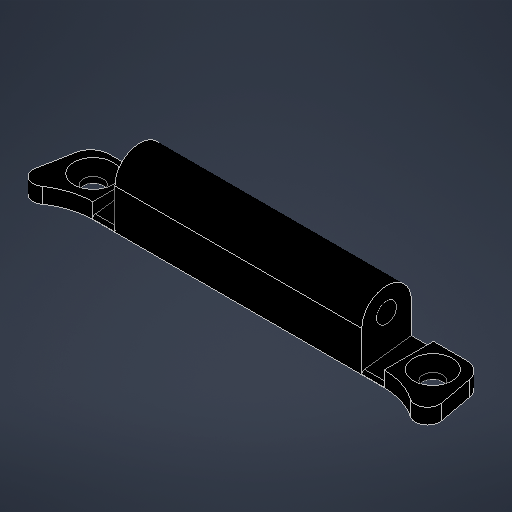
# Autodesk Inventor part: Dribbler Mount
Saved by Autodesk Inventor 2026.1 (Build 301233020, 233B)
## iProperties
Created: 2026-04-20
Part Number: Dribbler Mount
Material: Generic
Document SubType Name: Modeling
Designer: Bahaa
Mass: 3.13625 g
Surface Area: 24.6798 cm^2
Volume: 3.13625 cm^3
Density: 1 g/cm^3
Appearance: Black PLA
Author: Bahaa
Autodesk Inventor part; units mm, degrees
ref_plane "YZ Plane" through (0, 0, 0) normal (1, 0, 0) x (0, 1, 0)
ref_plane "XZ Plane" through (0, 0, 0) normal (0, 1, 0) x (-1, 0, 0)
ref_plane "XY Plane" through (0, 0, 0) normal (0, 0, 1) x (1, 0, 0)
sketch "Sketch1" plane through (0, 0, 0) normal (0, 0, 1) x (1, 0, 0)
  line L0 (-20, -4) -> (20, -4)
  line L1 (20, -4) -> (20, 4)
  line L2 (20, 4) -> (-20, 4)
  line L3 (-20, 4) -> (-20, -4)
  line L4 (-20, -4) -> (20, 4) construction
  line L5 (20, -4) -> (-20, 4) construction
  line L6 (-23.4, -4) -> (23.4, -4)
  line L7 (23.4, -4) -> (23.4, 4)
  line L8 (23.4, 4) -> (-23.4, 4)
  line L9 (-23.4, 4) -> (-23.4, -4)
  line L10 (-23.4, -4) -> (23.4, 4) construction
  line L11 (23.4, -4) -> (-23.4, 4) construction
  line L12 (-31.4, -4) -> (-23.4, -4)
  line L13 (-23.4, -4) -> (-23.4, 4)
  line L14 (-23.4, 4) -> (-28.9164, 4)
  line L15 (-31.4, 4) -> (-31.4, -4)
  circle A0 centre (-23.4, -15.5) radius 11.5
  line L16 (-31.8637, 1.5601) -> (-34.6978, -13.3529)
  line L17 (0, -4) -> (0, 4) construction
  circle A1 centre (23.4, -15.5) radius 11.5
  line L18 (31.8637, 1.5601) -> (34.6978, -13.3529)
  line L19 (31.4, -4) -> (23.4, -4)
  line L20 (23.4, 4) -> (28.9164, 4)
  line L21 (31.4, 4) -> (31.4, -4)
  line L22 (31.4, -4) -> (23.4, 4) construction
  line L23 (23.4, -4) -> (31.4, 4) construction
  arc A2 (-28.9164, 4) -> (-31.8637, 1.5601) centre (-28.9164, 1) ccw
  arc A3 (31.8637, 1.5601) -> (28.9164, 4) centre (28.9164, 1) ccw
  line L24 (23.4, -1.5) -> (-23.4, -1.5)
  line L25 (-20, 4) -> (-24, 4)
  line L26 (-24, 4) -> (-24, -4.0157)
  line L27 (-24, -4.0157) -> (-20, -4.0157)
  line L28 (-20, -4.0157) -> (-20, 4)
  line L29 (20, 4) -> (24, 4)
  line L30 (24, 4) -> (24, -4)
  line L31 (24, -4) -> (20, -4)
  line L32 (20, -4) -> (20, 4)
  point P0 (0, 0)
  point P1 (-20, 0)
  point P2 (-23.4, 0)
  point P3 (-27.5, 0)
  point P4 (27.5, 0)
  point P5 (23.4, -4)
  point P6 (-20, -1.5)
  point P7 (20, -1.5)
  point P8 (-31.4, 0)
  dimension "d0" = 40
  dimension "d1" = 8
  dimension "d3" = 3.4
  dimension "d4" = 8
  dimension "d5" = 8
  dimension "d6" = 0
  dimension "d7" = 11.5
  dimension "d8" = 23
  dimension "d11" = 3
  dimension "d31" = 5.5
  dimension "d35" = 27.5
  dimension "d40" = 4
  dimension "d41" = 4
  constraints: 62 end point, 10 midpoint, 10 parallel, 8 point on line, 7 symmetric about line, 6 perpendicular, 6 point on circle, 5 horizontal, 5 tangent, 3 centre point, 2 collinear, 1 equal radius, 1 horizontal alignment, 10 other
  measures "d0" distance of L2.end L1.end
  measures "d1" distance of L1.end L0.end
  measures "d3" distance of point (-20, 0) point (-23.4, 0)
  measures "d4" distance of L15.start L13.end
  measures "d5" distance of L15.start L12.start
  measures "d6" distance from line of L9 A0.centre
  measures "d7" vertical distance of L0.start A0.centre
  measures "d8" diameter of A0
  measures "d11" radius of A2
  measures "d31" distance from line of point (0, 4) L24
  measures "d35" distance of point (0, 0) point (-27.5, 0)
  measures "d40" distance of L27.end L26.end
  measures "d41" distance of L30.end L31.end
extrude "Extrusion1" add sketch "Sketch1" against normal blind 2.5 contours L3 L24 L1 L0 | L6 L9 L24 L3 | L1 L24 L7 L6 | L24 L9 L8 L3 | L3 L2 L1 L24 | L12 L26 L14 L9 | A0 L26 L12 | L1 L8 L7 L24 | L19 L21 A3 L18 A1 | L7 L20 L30 L19 | L26 A0 L16 A2 L15 L12 | L12 L15 A2 L14 L26 | L30 L20 A3 L21 L19
hole "Hole1" at (-27.5, 0, 0) at (27.5, 0, 0) direction (0, 0, -1) diameter 3.2 end through all countersink diameter 6.3 countersink angle 90 clearance for "Countersunk Flat Head Screw DIN EN ISO 2009" size "M3" standard "DIN"
fillet "Fillet1" radius 2 2 edges at (-34.6978, -13.3529, -1.25) (34.6978, -13.3529, -1.25)
extrude "Extrusion2" add sketch "Sketch1" along normal blind 8 contours L3 L24 L1 L0 | L3 L2 L1 L24
sketch "Sketch2" plane through (-20, -4, 0) normal (1, 0, 0) x (0, 0, -1)
  circle A0 centre (-4, 4) radius 4
  line L0 (-8, 8) -> (-8, 0) projected
  line L1 (2.5, 0) -> (2.5, 8) projected
  line L2 (2.5, 8) -> (0, 8) projected
  line L3 (0, 8) -> (-8, 8) projected
  line L4 (0, 0) -> (2.5, 0) projected
  line L5 (0, 0) -> (0, 8) projected
  line L6 (-8, 8) -> (-8, 0) projected
  line L7 (2, 0) -> (1, 8)
  line L8 (0, 2.5) -> (2.5, 2.5)
  line L9 (-8, 0) -> (0, 0) projected
  line L10 (0, 0) -> (-8, 0) projected
  line L11 (0, -2.3033) -> (2.5, -2.3033) projected
  line L12 (0, 8) -> (2, 8)
  line L13 (2, 8) -> (2, -2.3033)
  line L14 (2, -2.3033) -> (0, -2.3033)
  line L15 (0, -2.3033) -> (0, 8)
  line L16 (2.5, 0) -> (2.5, 8) projected
  line L17 (2.5, 8) -> (0, 8) projected
  line L18 (0, 8) -> (-8, 8) projected
  line L19 (-8, 8) -> (-8, 0) projected
  line L20 (-8, 0) -> (0, 0) projected
  line L21 (0, 0) -> (2.5, 0) projected
  line L22 (0, 0) -> (0, 8) projected
  line L23 (0, -2.3033) -> (2.5, -2.3033)
  line L24 (2.5, -2.3033) -> (2.5, 0)
  line L25 (2.5, 0) -> (0, 0)
  line L26 (0, 0) -> (0, -2.3033)
  circle A1 centre (-4.25, 4) radius 1.6
  point P0 (0, 4)
  point P1 (-4, 8)
  point P2 (-8, 4)
  point P3 (-8, 4)
  point P4 (0.6579, 6.9892)
  point P5 (1.4431, 1.9641)
  point P6 (1.6875, 2.5)
  point P7 (-4, 0)
  point P8 (0, 4)
  dimension "d27" = 0.5
  dimension "d36" = 1.5
  dimension "d42" = 3.2
  dimension "d43" = 4.25
  constraints: 20 end point, 4 parallel, 4 point on line, 3 perpendicular, 3 tangent, 2 centre point, 2 horizontal, 1 horizontal alignment, 1 midpoint
  measures "d27" distance from line of L1 L7.start
  measures "d36" distance of L1.end L7.end
  measures "d42" diameter of A1
  measures "d43" distance of point (0, 4) A1.centre
extrude "Extrusion3" cut sketch "Sketch2" along normal up to surface (40 mm away) contours A0 L0 L3 | L9 L0 A0 | A1
extrude "Extrusion4" cut sketch "Sketch2" against normal blind 3.6 contours L5 L2 L7 L8 | L8 L7 L4 L5 | L4 L13 L11 L15 | L4 L24 L11 L13
fillet "Fillet2" radius 0.5 1 edges at (-21.8, -4, -2)
mirror "Mirror1" about plane through (0, 0, 0) normal (1, 0, 0) of "Extrusion4", "Fillet2"
body "Solid1"
